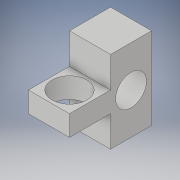
# Autodesk Inventor part: kamerahaltung
Saved by Autodesk Inventor 2018 (Build 220112000, 112)
## iProperties
Created: 2018-01-25
Part Number: kamerahaltung
Material: Generisch
Document SubType Name: Modeling
Designer: Andreas
Density: 1 g/cm^3
Appearance: Vorgabe
Author: Andreas
Autodesk Inventor part; units mm, degrees
ref_plane "YZ Plane" through (0, 0, 0) normal (1, 0, 0) x (0, 1, 0)
ref_plane "XZ Plane" through (0, 0, 0) normal (0, 1, 0) x (-1, 0, 0)
ref_plane "XY Plane" through (0, 0, 0) normal (0, 0, 1) x (1, 0, 0)
sketch "Skizze1" plane through (0, 0, 0) normal (0, 0, 1) x (1, 0, 0)
  line L0 (0, 0) -> (4, 0)
  line L1 (4, 0) -> (4, 8)
  line L2 (4, 8) -> (0, 8)
  line L3 (0, 8) -> (0, 0)
  dimension "d0" = 4
  dimension "d1" = 8
  constraints: 8 end point, 2 parallel, 1 horizontal, 1 perpendicular
  measures "d0" distance of L1.end L2.end
  measures "d1" distance of L0.end L1.end
extrude "Extrusion1" add sketch "Skizze1" against normal blind 8
sketch "Skizze12" plane through (4, 0, 0) normal (1, 0, 0) x (0, 0, -1)
  line L0 (0, 8) -> (0, 0) projected
  line L1 (0, 0) -> (3, 0)
  line L2 (3, 0) -> (3, 4)
  line L3 (3, 4) -> (0, 4)
  line L4 (0, 4) -> (0, 0)
  line L5 (8, 0) -> (5, 0)
  line L6 (5, 0) -> (5, 4)
  line L7 (5, 4) -> (8, 4)
  line L8 (8, 4) -> (8, 0)
  dimension "d45" = 4
  dimension "d46" = 4
  dimension "d47" = 3
  dimension "d48" = 3
  constraints: 16 end point, 4 parallel, 2 horizontal, 2 perpendicular
  measures "d45" distance of L7.end L5.start
  measures "d46" distance of L1.end L2.end
  measures "d47" distance of L2.end L3.end
  measures "d48" distance of L6.end L7.end
extrude "Extrusion10" cut sketch "Skizze12" against normal blind 5
sketch "Skizze13" plane through (4, 0, -3) normal (0, 0, 1) x (1, 0, 0)
  circle A0 centre (-2, 2) radius 1.7
  line L0 (0, 0) -> (-4, 0) projected
  line L1 (0, 4) -> (0, 0) projected
  dimension "d51" = 3.4
  dimension "d52" = 2
  dimension "d53" = 2
  constraints: 1 centre point
  measures "d51" diameter of A0
  measures "d52" distance from line of L0 A0.centre
  measures "d53" distance from line of L1 A0.centre
extrude "Extrusion11" cut sketch "Skizze13" against normal blind 3
sketch "Skizze14" plane through (4, 8, 0) normal (1, 0, 0) x (0, 0, -1)
  circle A0 centre (4, -2) radius 1.5
  line L0 (0, -4) -> (0, 0) projected
  line L1 (0, -4) -> (3, -4) projected
  point P0 (0, -8)
  dimension "d56" = 3
  dimension "d57" = 4
  dimension "d58" = 2
  constraints: 1 centre point
  measures "d56" diameter of A0
  measures "d57" distance from line of L0 A0.centre
  measures "d58" distance from line of L1 A0.centre
extrude "Extrusion12" cut sketch "Skizze14" against normal blind 10
